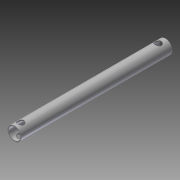
# Autodesk Inventor part: Horizantal Rod
Saved by Autodesk Inventor 2013 (Build 170138000, 138)
## iProperties
Created: 2014-05-22
Part Number: Horizantal Rod
Material: Steel
Document SubType Name: Modeling
Designer: nojessen
Mass: 308.401 g
Surface Area: 415.272 cm^2
Volume: 39.2868 cm^3
Density: 7.85 g/cm^3
Author: nojessen
Autodesk Inventor part; units mm, degrees
ref_plane "YZ Plane" through (0, 0, 0) normal (1, 0, 0) x (0, 1, 0)
ref_plane "XZ Plane" through (0, 0, 0) normal (0, 1, 0) x (-1, 0, 0)
ref_plane "XY Plane" through (0, 0, 0) normal (0, 0, 1) x (1, 0, 0)
sketch "Sketch1" plane through (0, 0, 0) normal (0, 0, 1) x (1, 0, 0)
  circle A0 centre (0, 0) radius 12.7
  circle A1 centre (0, 0) radius 10.795
  line L0 (0, 0) -> (12.7, 0)
  dimension "d0" = 25.4
  dimension "d1" = 21.59
  constraints: 2 coincident, 2 end point, 1 centre point, 1 horizontal, 1 horizontal alignment, 2 other
  measures "d1" diameter of A1
extrude "Extrusion1" add sketch "Sketch1" along normal blind 279.4
ref_plane "Work Plane2" through (0, 12.7, 0) normal (0, 1, 0) x (1, 0, 0)
ref_plane "Work Plane1" through (0, 0, 0) normal (0, 1, 0) x (1, 0, 0)
sketch "Sketch2" plane through (0, 12.7, 0) normal (0, 1, 0) x (1, 0, 0)
  line L0 (0, 0) -> (0, -279.4)
  line L1 (0, -279.4) -> (0, -267.97)
  circle A0 centre (0, -267.97) radius 6.35
  line L2 (0, 0) -> (0, -13.97)
  circle A1 centre (0, -13.97) radius 6.35
  dimension "d6" = 279.4
  dimension "d7" = 11.43
  dimension "d8" = 12.7
  dimension "d9" = 13.97
  dimension "d10" = 12.7
  constraints: 6 end point, 2 centre point, 2 coincident, 2 point on line, 1 vertical
  measures "d6" distance of L0.start L0.end
  measures "d7" distance of L0.end L1.end
  measures "d8" diameter of A0
  measures "d9" distance of L0.start L2.end
  measures "d10" diameter of A1
extrude "Extrusion2" cut sketch "Sketch2" against normal blind 279.4
body "Solid1"
